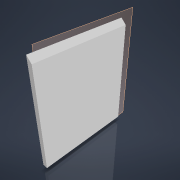
# Autodesk Inventor part: N__side_sticker
Saved by Autodesk Inventor 2022 (Build 260153070, 153G)
## iProperties
Created: 2021-11-16
Part Number: N__side_sticker
Material: Типовые
Document SubType Name: Modeling
Designer: kalugin_a
Density: 1 g/cm^3
Appearance: По умолчанию
Author: kalugin_a
Autodesk Inventor part; units mm, degrees
ref_plane "YZ Plane" through (0, 0, 0) normal (1, 0, 0) x (0, 1, 0)
ref_plane "XZ Plane" through (0, 0, 0) normal (0, 1, 0) x (-1, 0, 0)
ref_plane "XY Plane" through (0, 0, 0) normal (0, 0, 1) x (1, 0, 0)
ref_plane "РабПлоскость1" through (203.4395, -285.3633, -641.5751) normal (1, 0, 0) x (0, 1, 0)
sketch "Эскиз1" plane through (203.4395, -285.3633, -641.5751) normal (1, 0, 0) x (0, 1, 0)
  line L0 (-170.5002, 182.8495) -> (170.5001, 182.8495)
  line L1 (170.5001, 182.8495) -> (170.5001, -151.0964)
  line L2 (170.5001, -151.0964) -> (-170.5002, -151.0964)
  line L3 (-170.5002, -151.0964) -> (-170.5002, 182.8495)
  point P0 (285.3633, 641.5751)
  constraints: 8 end point, 2 parallel, 1 horizontal, 1 perpendicular
extrude "Выдавливание1" add sketch "Эскиз1" along normal blind 16
chamfer "Фаска1" distance 16 angle 45 1 edges at (219.4395, -114.8632, -625.6985)
